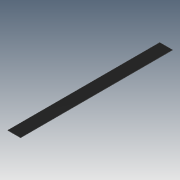
# Autodesk Inventor part: GE-12022-01
Saved by Autodesk Inventor 2012 (Build 160160000, 160)
## iProperties
Created: 2011-06-06
Part Number: GE-12022-01
Document SubType Name: Modeling
Designer: dfoster
Density: 7.85 g/cm^3
Material: Steel
Mass: 15023.8 g
Surface Area: 8423.68 cm^2
Volume: 1913.86 cm^3
Description: 4" Hook Velcro, Adhesive Backed
Title: 4" Hook Velcro, Adhesive Backed
Author: dfoster
Autodesk Inventor part; units mm, degrees
ref_plane "YZ Plane" through (0, 0, 0) normal (1, 0, 0) x (0, 1, 0)
ref_plane "XZ Plane" through (0, 0, 0) normal (0, 1, 0) x (-1, 0, 0)
ref_plane "XY Plane" through (0, 0, 0) normal (0, 0, 1) x (1, 0, 0)
sketch "Sketch1" plane through (0, 0, 0) normal (0, 0, 1) x (1, 0, 0)
  line L0 (-119.8515, -15.2817) -> (-18.2515, -15.2817)
  line L1 (-18.2515, -13.3767) -> (-119.8515, -13.3767)
  line L2 (-119.8515, -13.3767) -> (-119.8515, -15.2817)
  line L3 (-18.2515, -13.3767) -> (-18.2515, -15.2817)
  dimension "d63" = 101.6
  dimension "d64" = 1.905
  constraints: 8 end point, 1 horizontal, 1 parallel, 1 vertical
  measures "d63" distance of L1.start L1.end
  measures "d64" distance between parallel lines of L0 L1
extrude "Extrusion1" add sketch "Sketch1" along normal blind 1206.5
body "Solid1"
